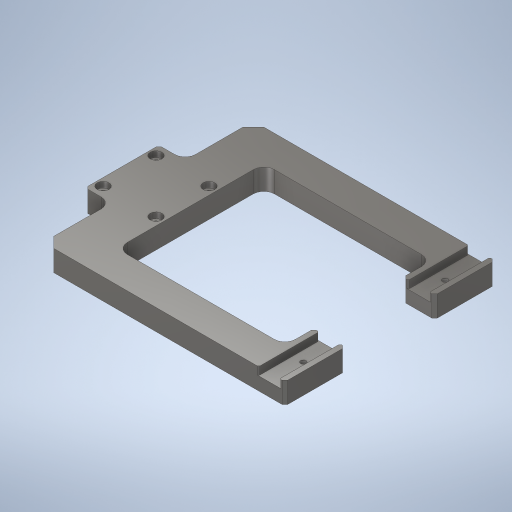
# Autodesk Inventor part: Holder - headbars - L - LH
Saved by Autodesk Inventor 2023 (Build 270158000, 158)
## iProperties
Created: 2019-01-08
Part Number: Holder - headbars - L - LH
Material: Stainless Steel
Document SubType Name: Modeling
Designer: Tanya
Density: 8 g/cm^3
Appearance: Semi-Polished
Author: Tanya
Autodesk Inventor part; units mm, degrees
ref_plane "YZ Plane" through (0, 0, 0) normal (1, 0, 0) x (0, 1, 0)
sketch "Sketch1" plane through (0, 0, 0) normal (0, 1, 0) x (-1, 0, 0)
  line L0 (0, -88.9) -> (0, 88.9) projected
  line L1 (-102.235, 0) -> (124.46, 0) projected
  line L2 (50.8, 44.45) -> (-50.8, 44.45)
  line L3 (-50.8, -44.45) -> (50.8, -44.45)
  line L4 (50.8, -44.45) -> (50.8, 44.45)
  line L5 (76.2, 63.5) -> (-69.85, 63.5)
  line L6 (-69.85, -63.5) -> (76.2, -63.5)
  line L7 (76.2, -63.5) -> (76.2, 63.5)
  line L8 (-50.8, 26.9875) -> (-69.85, 26.9875)
  line L9 (-69.85, -26.9875) -> (-50.8, -26.9875)
  line L10 (-50.8, 44.45) -> (-50.8, 26.9875)
  line L11 (-50.8, -26.9875) -> (-50.8, -44.45)
  line L12 (-69.85, 63.5) -> (-69.85, 26.9875)
  line L13 (-69.85, -26.9875) -> (-69.85, -63.5)
  line L14 (-53.975, 63.5) -> (-66.675, 63.5) construction
  line L15 (-66.675, 63.5) -> (-66.675, 26.9875) construction
  line L16 (-66.675, 26.9875) -> (-53.975, 26.9875) construction
  line L17 (-53.975, 26.9875) -> (-53.975, 63.5) construction
  line L18 (-53.975, -26.9875) -> (-66.675, -26.9875) construction
  line L19 (-66.675, -26.9875) -> (-66.675, -63.5) construction
  line L20 (-66.675, -63.5) -> (-53.975, -63.5) construction
  line L21 (-53.975, -63.5) -> (-53.975, -26.9875) construction
  line L22 (-60.325, 63.5) -> (-60.325, 26.9875) construction
  line L23 (-60.325, -26.9875) -> (-60.325, -63.5) construction
  line L24 (76.2, 22.225) -> (92.075, 22.225)
  line L25 (92.075, 22.225) -> (92.075, -22.225)
  line L26 (92.075, -22.225) -> (76.2, -22.225)
  line L27 (76.2, -22.225) -> (76.2, 22.225)
  point P0 (0, 0)
  dimension "d0" = 12.7
  dimension "d1" = 136.525
  dimension "d2" = 53.975
  dimension "d3" = 26.9875
  dimension "d4" = 101.6
  dimension "d5" = 19.05
  dimension "d6" = 3.175
  dimension "d7" = 50.8
  dimension "d8" = 88.9
  dimension "d9" = 44.45
  dimension "d10" = 19.05
  dimension "d11" = 19.05
  dimension "d24" = 25.4
  dimension "d25" = 44.45
  dimension "d26" = 22.225
  dimension "d27" = 41.275
  constraints: 52 end point, 13 parallel, 7 perpendicular, 6 horizontal, 5 point on line, 4 collinear, 4 midpoint
  measures "d0" distance between parallel lines of L15 L17
  measures "d1" distance from line of L22.start L7
  measures "d2" distance between parallel lines of L9 L8
  measures "d3" distance between parallel lines of L1 L9
  measures "d4" distance between parallel lines of L11 L4
  measures "d5" distance between parallel lines of L13 L11
  measures "d6" distance between parallel lines of L13 L19
  measures "d7" distance between parallel lines of L0 L11
  measures "d8" distance between parallel lines of L3 L2
  measures "d9" distance between parallel lines of L3 L1
  measures "d10" distance between parallel lines of L5 L2
  measures "d11" distance between parallel lines of L6 L3
  measures "d24" distance between parallel lines of L4 L7
  measures "d25" distance of L24.end L25.end
  measures "d26" distance between parallel lines of L26 L1
  measures "d27" distance between parallel lines of L25 L4
extrude "Extrusion1" add sketch "Sketch1" along normal mid plane 12.7 contours L6 L13 L9 L11 L3 L0 | L0 L3 L4 L1 L7 L6 | L7 L1 L25 L26 | L2 L10 L8 L12 L5 L0 | L0 L5 L7 L1 L4 L2 | L7 L24 L25 L1
sketch "Sketch2" plane through (0, 6.35, 0) normal (0, 1, 0) x (1, 0, 0)
  line L0 (50.8, -44.45) -> (-50.8, -44.45) projected
  line L1 (-50.8, -44.45) -> (-50.8, 44.45) projected
  line L2 (-50.8, 44.45) -> (50.8, 44.45) projected
  line L3 (50.8, 44.45) -> (50.8, 26.9875) projected
  line L4 (50.8, 26.9875) -> (69.85, 26.9875) projected
  line L5 (69.85, 26.9875) -> (69.85, 63.5) projected
  line L6 (69.85, 63.5) -> (-76.2, 63.5) projected
  line L7 (-76.2, -22.225) -> (-76.2, -63.5) projected
  line L8 (-76.2, -63.5) -> (69.85, -63.5) projected
  line L9 (69.85, -63.5) -> (69.85, -26.9875) projected
  line L10 (69.85, -26.9875) -> (50.8, -26.9875) projected
  line L11 (50.8, -26.9875) -> (50.8, -44.45) projected
  line L12 (-76.2, -63.5) -> (69.85, -63.5) projected
  line L13 (53.975, -63.5) -> (66.675, -63.5)
  line L14 (66.675, -63.5) -> (66.675, -26.9875)
  line L15 (66.675, -26.9875) -> (53.975, -26.9875)
  line L16 (53.975, -26.9875) -> (53.975, -63.5)
  line L17 (50.8, 26.9875) -> (69.85, 26.9875) projected
  line L18 (69.85, 63.5) -> (-76.2, 63.5) projected
  line L19 (53.975, 26.9875) -> (66.675, 26.9875)
  line L20 (66.675, 26.9875) -> (66.675, 63.5)
  line L21 (66.675, 63.5) -> (53.975, 63.5)
  line L22 (53.975, 63.5) -> (53.975, 26.9875)
  line L23 (60.325, -63.5) -> (60.325, 99.2856) construction
  line L24 (102.235, 0) -> (-124.46, 0) projected
  line L25 (-76.2, 22.225) -> (-92.075, 22.225) projected
  line L26 (-92.075, 22.225) -> (-92.075, -22.225) projected
  line L27 (-92.075, -22.225) -> (-76.2, -22.225) projected
  line L28 (-76.2, 63.5) -> (-76.2, 22.225) projected
  point P0 (0, 0)
  dimension "d14" = 12.7
  dimension "d15" = 6.35
  dimension "d16" = 19.05
  dimension "d17" = 3.175
  constraints: 18 end point, 5 parallel, 5 point on line, 2 horizontal, 2 perpendicular, 1 collinear, 1 midpoint
  measures "d14" distance between parallel lines of L16 L14
  measures "d15" distance between parallel lines of L14 L23
  measures "d16" distance between parallel lines of L9 L11
  measures "d17" distance between parallel lines of L14 L9
extrude "Extrusion2" cut sketch "Sketch2" against normal blind 4.7625 contours L10 L14 L8 L16 | L22 L6 L20 L4
sketch "Sketch3" plane through (0, 6.35, 0) normal (0, 1, 0) x (1, 0, 0)
  line L0 (-50.8, 12.4641) -> (-90.8, 12.4641) projected
  line L1 (102.235, 0) -> (-124.46, 0) projected
  line L2 (53.975, -63.5) -> (53.975, -26.9875) projected
  line L3 (53.975, -26.9875) -> (50.8, -26.9875) projected
  line L4 (50.8, -26.9875) -> (50.8, -44.45) projected
  line L5 (50.8, -44.45) -> (-50.8, -44.45) projected
  line L6 (-50.8, -44.45) -> (-50.8, 44.45) projected
  line L7 (-50.8, 44.45) -> (50.8, 44.45) projected
  line L8 (50.8, 44.45) -> (50.8, 26.9875) projected
  line L9 (50.8, 26.9875) -> (53.975, 26.9875) projected
  line L10 (53.975, 26.9875) -> (53.975, 63.5) projected
  line L11 (53.975, 63.5) -> (-76.2, 63.5) projected
  line L12 (-76.2, -22.225) -> (-76.2, -63.5) projected
  line L13 (-76.2, -63.5) -> (53.975, -63.5) projected
  line L14 (-76.2, 63.5) -> (-76.2, 22.225) projected
  line L15 (-76.2, 22.225) -> (-92.075, 22.225) projected
  line L16 (-92.075, 22.225) -> (-92.075, -22.225) projected
  line L17 (-92.075, -22.225) -> (-76.2, -22.225) projected
  point P0 (0, 0)
  point P1 (-87.5625, 16)
  point P2 (-55.5625, 16)
  point P3 (-55.5625, -16)
  point P4 (-87.5625, -16)
  dimension "d20" = 32
  dimension "d21" = 32
  dimension "d22" = 16
  dimension "d23" = 4.7625
  constraints: 2 horizontal alignment, 2 vertical alignment
  measures "d20" distance of point (-55.562, -16) point (-87.562, -16)
  measures "d21" distance of point (-55.562, -16) point (-55.562, 16)
  measures "d22" distance from line of L1 point (-55.562, 16)
  measures "d23" distance from line of point (-55.562, -16) L6
hole "Hole1" at (-87.5625, 6.35, -16) at (-55.5625, 6.35, -16) at (-55.5625, 6.35, 16) at (-87.5625, 6.35, 16) direction (0, -1, 0) diameter 3.81 end through all counterbore diameter 7.1374 counterbore depth 3.5052 clearance for "Socket Head Cap Screw" size "#6" standard "Ansi Unified Screw Threads"
fillet "Fillet1" radius 6.35 6 edges at (-76.2, 0, 22.225) (-76.2, 0, -22.225) (-50.8, 0, -44.45) (-50.8, 0, 44.45) (50.8, 0, 44.45) (50.8, 0, -44.45)
chamfer "Chamfer1" distance 1.5875 angle 45 8 edges at (-92.075, 0, 22.225) (-92.075, 0, -22.225) (69.85, 0, 26.9875) (50.8, 0, 26.9875) (69.85, 0, 63.5) (69.85, 0, -26.9875) (69.85, 0, -63.5) (50.8, 0, -26.9875)
chamfer "Chamfer2" distance 6.35 angle 45 2 edges at (-76.2, 0, 63.5) (-76.2, 0, -63.5)
ref_plane "Work Plane1" through (60.325, 6.35, 63.5) normal (1, 0, 0) x (0, 0, -1)
ref_plane "Work Plane2" through (60.325, 6.35, -26.9875) normal (1, 0, 0) x (0, 0, -1)
sketch "Sketch4" plane through (0, 1.5875, 0) normal (0, 1, 0) x (1, 0, 0)
  line L0 (53.975, 63.5) -> (66.675, 63.5) projected
  line L1 (53.975, 26.9875) -> (53.975, 63.5) projected
  line L2 (66.675, 26.9875) -> (53.975, 26.9875) projected
  line L3 (66.675, 63.5) -> (66.675, 26.9875) projected
  line L4 (53.975, -26.9875) -> (66.675, -26.9875) projected
  line L5 (53.975, -63.5) -> (53.975, -26.9875) projected
  line L6 (66.675, -63.5) -> (53.975, -63.5) projected
  line L7 (66.675, -26.9875) -> (66.675, -63.5) projected
  point P0 (0, 0)
  point P1 (60.325, 42.8625)
  point P2 (60.325, -42.8625)
  dimension "d44" = 15.875
  dimension "d45" = 15.875
  dimension "d46" = 6.35
  constraints: 1 vertical alignment
  measures "d44" distance from line of point (60.325, 42.862) L2
  measures "d45" distance from line of L4 point (60.325, -42.863)
  measures "d46" distance from line of point (60.325, 42.862) L3
hole "Hole2" at (60.325, 1.5875, -42.8625) at (60.325, 1.5875, 42.8625) direction (0, -1, 0) diameter 3.302 end through all thread size "8-32 UNC" class "2B" standard "ANSI Unified Screw Threads"
chamfer "Chamfer3" distance 0.7937 angle 45 8 edges at (53.975, 3.9687, 63.5) (66.675, 3.9687, 63.5) (53.975, 3.9687, 26.9875) (66.675, 3.9687, 26.9875) (53.975, 3.9687, -26.9875) (66.675, 3.9687, -26.9875) (53.975, 3.9687, -63.5) (66.675, 3.9687, -63.5)
equation "\"d3\" = 0.5 * d2"
equation "\"d7\" = 0.5 * d4"
equation "\"d9\" = 0.5 * d8"
equation "\"d11\" = d10"
equation "\"d26\" = 0.5 * d25"
equation "\"d21\" = d20"
equation "\"d22\" = 0.5 * d21"
equation "\"d45\" = d44"
body "Solid1"
